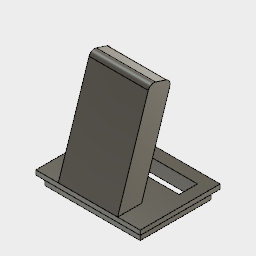
Jenkins_Monitor_Top_LCD_Insert v1 (Autodesk Fusion 360 design; units mm, degrees)
Autodesk Fusion 360 part; units mm, degrees
sketch "Sketch1" plane through (0, 0, 0) normal (0, 0, 1) x (1, 0, 0)
  line L0 (-20.9, 15.55) -> (20.9, 15.55)
  line L1 (20.9, 15.55) -> (20.9, -15.55)
  line L2 (20.9, -15.55) -> (-20.9, -15.55)
  line L3 (-20.9, -15.55) -> (-20.9, 15.55)
  line L4 (-20.9, 15.55) -> (20.9, -15.55) construction
  line L5 (20.9, 15.55) -> (-20.9, -15.55) construction
  line L6 (-22.9, 17.55) -> (22.9, 17.55)
  line L7 (22.9, 17.55) -> (22.9, -17.55)
  line L8 (22.9, -17.55) -> (-22.9, -17.55)
  line L9 (-22.9, -17.55) -> (-22.9, 17.55)
  line L10 (-22.9, 17.55) -> (22.9, -17.55) construction
  line L11 (22.9, 17.55) -> (-22.9, -17.55) construction
  line L12 (0, 15.55) -> (0, 12.55)
  line L13 (0, 12.55) -> (17.9, 12.55)
  line L14 (17.9, 12.55) -> (-17.9, 12.55)
  line L15 (-17.9, 12.55) -> (-17.9, 4.55)
  line L16 (-17.9, 4.55) -> (17.9, 4.55)
  line L17 (17.9, 4.55) -> (17.9, 12.55)
  dimension "d1" = 41.8
  dimension "d2" = 31.1
  dimension "d3" = 45.8
  dimension "d4" = 35.1
  dimension "d16" = 3
  dimension "d17" = 17.9
  dimension "d18" = 35.8
  dimension "d19" = 8
  measures "d1" distance of L1.end L2.end
  measures "d2" distance of L0.end L1.end
  measures "d3" distance of L7.end L8.end
  measures "d4" distance of L6.end L7.end
  measures "d16" distance of L12.start L12.end
  measures "d17" distance of L12.end L13.end
  measures "d18" distance of L13.end L14.end
  measures "d19" distance of L13.end L16.end
extrude "Extrude1" add sketch "Sketch1" along normal blind 6 contours L0 L1 L2 L3 | L6 L7 L8 L9 | L13 L14 L15 L16 L17
extrude "Extrude2" cut sketch "Sketch1" along normal blind 4 contours L6 L7 L8 L9
ref_plane "WorkPlane1" through (0, -17.55, 6) normal (0, 0.309017, 0.951057) x (1, 0, 0)
sketch "Sketch2" plane through (0, -17.55, 6) normal (0, 0.309017, 0.951057) x (1, 0, 0)
  line L0 (0, 0) -> (-13, 0)
  line L1 (-13, 0) -> (13, 0)
  line L2 (13, 0) -> (13, 10)
  line L3 (13, 10) -> (-13, 10)
  line L4 (-13, 10) -> (-13, 0)
  dimension "d10" = 13
  dimension "d11" = 26
  dimension "d12" = 10
  measures "d10" distance of L0.start L0.end
  measures "d11" distance of L0.end L1.end
  measures "d12" distance of L0.end L3.end
extrude "Extrude3" add sketch "Sketch2" along normal blind 46
fillet "Fillet1" radius 2.5 2 edges at (0, 6.1753, 46.6584) (0, -3.3352, 49.7486)
extrude "Extrude4" cut sketch "Sketch1" along normal up to surface (6 mm away) contours L13 L14 L15 L16 L17
equation "d17 = ( 41.8 / 2 ) * 1 mm - 3 mm"
equation "d18 = ( 17.9 * 2 ) * 1 mm"
